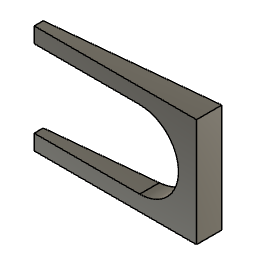
Delta Shower handle removal wedges (Autodesk Fusion 360 design; units mm, degrees)
Autodesk Fusion 360 part; units mm, degrees
sketch "Sketch1" plane through (0, 0, 0) normal (0, 0, 1) x (1, 0, 0)
  line L0 (0, 0) -> (90, 0)
  line L1 (90, 0) -> (90, 14)
  line L2 (90, 14) -> (0, 5)
  line L3 (0, 5) -> (0, 0)
  dimension "d1" = 5
  dimension "d2" = 14
  dimension "d3" = 90
  constraint coincident L0.start L3.end
  constraint horizontal L0
  constraint perpendicular L0 L1
  constraint perpendicular L0 L3
  measures "d1" distance of L2.end L0.start
  measures "d2" distance of L0.end L1.end
  measures "d3" distance of L0.start L0.end
extrude "Extrude1" add sketch "Sketch1" along normal blind 60
sketch "Sketch2" plane through (0, 0, 0) normal (0, -1, 0) x (1, 0, 0)
  line L0 (0, 0) -> (90, 0)
  line L1 (90, 0) -> (90, 60)
  line L2 (90, 60) -> (0, 60)
  line L3 (0, 60) -> (0, 0)
  line L4 (0, 30) -> (90, 30) construction
  line L5 (58.5, 51.5) -> (0, 51.5)
  line L6 (58.5, 8.5) -> (0, 8.5)
  arc A0 (58.5, 8.5) -> (58.5, 51.5) centre (58.5, 30) ccw
  dimension "d6" = 43
  dimension "d8" = 10
  constraint midpoint L3 L4.start
  constraint midpoint L1 L4.end
  constraint coincident A0.centre L4
  constraint coincident L3 L5.end
  constraint tangent L5 A0
  constraint horizontal L5
  constraint symmetric L4 L5.start L6.start
  constraint symmetric L4 L5.end L6.end
  measures "d6" diameter of A0
  measures "d8" distance of L4.end A0
extrude "Extrude2" cut sketch "Sketch2" against normal blind 46.857 contours L3 L5 L6 A0
named bodies: "Wedge"
